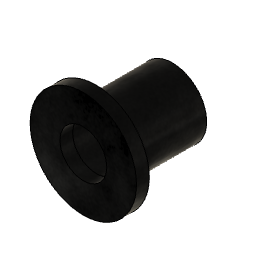
aa FINAL MODEL (Autodesk Fusion 360 archive; units mm, degrees)
design "Black bolt filler for flange"
Autodesk Fusion 360 part; units mm, degrees
note: some values were not read from the file. Chosen so that the rebuilt part matches the saved one: which bodies a step acts on; which face or edge a step refers to; how an offset face is resized.
sketch "Sketch1" plane through (0, 0, 0) normal (0, 1, 0) x (1, 0, 0)
  circle A0 centre (0, 0) radius 12.5
  dimension "d1" = 25
  constraint coincident A0.centre origin
  measures "d1" diameter of A0
extrude "Extrude1" add sketch "Sketch1" along normal blind 3 makes body 1
cylinder "CylinderPrimitive1" add diameter 16 height 18 placed x (1, 0, 0) y (0, 0, -1) z (0, 1, 0) at (0, 3, 0) separate body makes body 2
cylinder "CylinderPrimitive2" cut diameter 11 height -30 placed x (1, 0, 0) y (0, 0, -1) z (0, 1, 0) at (0, 21, 0) bodies 1 2

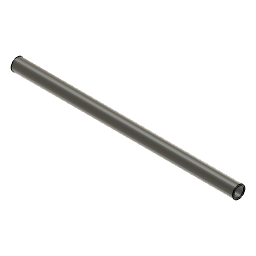
design "Pipe F"
Autodesk Fusion 360 part; units mm, degrees
sketch "Sketch1" plane through (0, 0, 0) normal (0, 1, 0) x (1, 0, 0)
  line L0 (-120, 0) -> (743.6, 0)
  dimension "d1" = 863.6
  constraint horizontal L0
  measures "d1" distance of L0.start L0.end
pipe "Pipe1" add diameter 48 wall 5 path "Sketch1" along L0

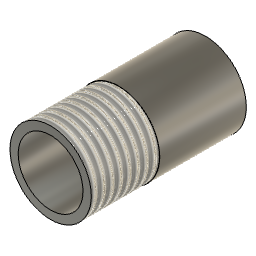
design "Short Piece for Tube"
Autodesk Fusion 360 part; units mm, degrees
sketch "Sketch1" plane through (0, 0, 0) normal (0, 1, 0) x (1, 0, 0)
  circle A0 centre (0, 0) radius 24
  circle A1 centre (0, 0) radius 19
  dimension "d1" = 48
  dimension "d2" = 38
  constraint coincident A0.centre A1.centre
  measures "d1" diameter of A0
  measures "d2" diameter of A1
extrude "Extrude1" add sketch "Sketch1" along normal blind 50.8 makes body 1
sketch "Sketch2" plane through (0, 0, 0) normal (0, -1, 0) x (1, 0, 0)
  circle A0 centre (0, 0) radius 19
  circle A1 centre (0, 0) radius 24
  circle A2 centre (0, 0) radius 24
  circle A3 centre (0, 0) radius 19
  dimension "d5" = 48
  dimension "d6" = 38
  constraint coincident A0.centre A1.centre
  measures "d5" diameter of A2
  measures "d6" diameter of A3
extrude "Extrude2" add sketch "Sketch2" along normal blind 40 bodies 1
sketch "Sketch4" plane through (0, 0, 0) normal (1, 0, 0) x (0, 1, 0)
  line L0 (0, 27) -> (0, -28)
  line L1 (-40, 24) -> (-40, -24)
  dimension "d10" = 40
  constraint vertical L0
  measures "d10" distance of L0 L1
split "Split2" by curves path "Sketch4" along L0 bodies 1 makes body 2 at (23.8807, -13.3333, -2.3896)
thread "Thread1" "ISO Metric profile 48.0 M48x5 M48x5 6g" major diameter 47.664 minor diameter 41.9335 pitch 5 angle 60 resizes the face on face at (23.8807, -13.3333, -2.3896) on bodies 2

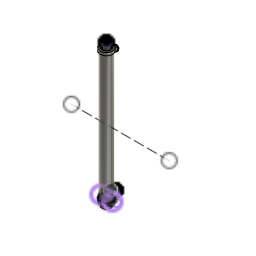
design "Heat Exchange"
Autodesk Fusion 360 part; units mm, degrees
sketch "Sketch1" plane through (0, 0, 0) normal (0, 0, 1) x (1, 0, 0)
  circle A0 centre (0, 0) radius 40
  dimension "d1" = 80
  constraint coincident A0.centre origin
  measures "d1" diameter of A0
extrude "Extrude1" add sketch "Sketch1" along normal blind 914.4 makes body 1
sketch "Sketch2" plane through (0, 0, 914.4) normal (0, 0, 1) x (-1, 0, 0)
  circle A0 centre (0, 0) radius 40
  circle A1 centre (0, 0) radius 44.45
  dimension "d4" = 88.9
  constraint concentric A0 A1
  measures "d4" diameter of A1
extrude "Extrude2" add sketch "Sketch2" along normal blind 20 contours A0 | A1 bodies 1
sketch "Sketch3" plane through (0, 0, 934.4) normal (0, 0, 1) x (-1, 0, 0)
  circle A0 centre (0, 0) radius 44.45
  circle A1 centre (0, 0) radius 29.5
  dimension "d7" = 59
  constraint coincident A0.centre A1.centre
  measures "d7" diameter of A1
extrude "Extrude3" add sketch "Sketch3" along normal blind 31 contours A1 bodies 1
sketch "Sketch4" plane through (0, 0, 965.4) normal (0, 0, 1) x (-1, 0, 0)
  circle A0 centre (0, 0) radius 29.5
  circle A1 centre (0, 0) radius 24
  dimension "d10" = 48
  constraint coincident A0.centre A1.centre
  measures "d10" diameter of A1
extrude "Extrude4" cut sketch "Sketch4" against normal blind 30 contours A1 bodies 1
sketch "Sketch6" plane through (0, 0, 0) normal (0, 0, -1) x (1, 0, 0)
  circle A0 centre (0, 0) radius 40
  circle A1 centre (0, 0) radius 44.45
  dimension "d15" = 88.9
  constraint coincident A0.centre A1.centre
  measures "d15" diameter of A1
extrude "Extrude5" add sketch "Sketch6" along normal blind 20 contours A0 | A1 bodies 1
sketch "Sketch7" plane through (0, 0, -20) normal (0, 0, -1) x (1, 0, 0)
  circle A0 centre (0, 0) radius 44.45
  circle A1 centre (0, 0) radius 22.55
  dimension "d18" = 45.1
  constraint concentric A0 A1
  measures "d18" diameter of A1
ref_plane "WorkPlane2" through (0, 29, 0) normal (0, 1, 0) x (0, 0, 1)
sketch "Sketch10" plane through (0, 29, 0) normal (0, 1, 0) x (1, 0, 0)
  line L0 (22.25, -14.95) -> (22.25, 7.3)
  line L1 (22.25, 7.3) -> (-22.25, 7.3)
  line L2 (-22.25, 7.3) -> (-22.25, -14.95)
  arc A0 (-22.25, -14.95) -> (22.25, -14.95) centre (0, -14.95) ccw
  line L3 (44.45, 20) -> (-44.45, 20)
  point P0 (0, -37.2)
  dimension "d27" = 44.5
  dimension "d28" = 44.5
  dimension "d30" = 12.7
  constraint vertical L0
  constraint perpendicular L0 L1
  constraint perpendicular L1 L2
  constraint tangent L2 A0
  constraint tangent L0 A0
  constraint midpoint A0 P0
  constraint vertical origin A0.centre
  measures "d27" distance of L0.end L1.end
  measures "d28" distance of L1 P0
  measures "d30" distance of L1 L3
extrude "Extrude8" add sketch "Sketch10" along normal blind 28.575 bodies 1
sketch "Sketch11" plane through (0, 57.575, 0) normal (0, 1, 0) x (-1, 0, 0)
  arc A0 (22.25, 14.95) -> (-22.25, 14.95) centre (0, 14.95) ccw
  line L0 (-22.25, 14.95) -> (-22.25, -7.3)
  line L1 (-22.25, -7.3) -> (22.25, -7.3)
  line L2 (22.25, -7.3) -> (22.25, 14.95)
  circle A1 centre (0, 14.95) radius 16
  dimension "d33" = 32
  constraint coincident A0.centre A1.centre
  measures "d33" diameter of A1
extrude "Extrude9" add sketch "Sketch11" along normal blind 5 contours A1 bodies 1
sketch "Sketch12" plane through (0, 0, 0) normal (0, 1, 0) x (1, 0, 0)
  line L0 (450, -457.2) -> (-250, -457.2) construction
  line L1 (44.45, 0) -> (-44.45, 0) construction
  dimension "d36" = 457.2
  constraint horizontal L0
  measures "d36" distance of L0 L1
ref_plane "WorkPlane3" through (0, 0, 458) normal (0, 0, 1) x (1, 0, 0)
mirror "Mirror1" about plane through (0, 0, 458) normal (0, 0, 1) of "Extrude8"
sketch "Sketch13" plane through (0, 62.575, 0) normal (0, 1, 0) x (-1, 0, 0)
  circle A0 centre (0, 14.95) radius 16
  line L0 (0.261, 38.0425) -> (-19.8682, 26.7223)
  line L1 (-19.8682, 26.7223) -> (-20.1292, 3.6298)
  line L2 (-20.1292, 3.6298) -> (-0.261, -8.1425)
  line L3 (-0.261, -8.1425) -> (19.8682, 3.1777)
  line L4 (19.8682, 3.1777) -> (20.1292, 26.2702)
  line L5 (20.1292, 26.2702) -> (0.261, 38.0425)
  point P0 (0, 14.95)
  dimension "d42" = 20
  constraint coincident P0 A0.centre
  measures "d42" distance of P0 L5
extrude "Extrude10" add sketch "Sketch13" along normal blind 4 separate body makes body 2
extrude "Extrude11" add 1 faces at (3.6165, 62.575, 23.0058) along direction (0, 1, 0) blind 7 on bodies 1 bodies 1 2
sketch "Sketch15" plane through (0, 69.575, 0) normal (0, 1, 0) x (-1, 0, 0)
  circle A0 centre (0, 14.95) radius 16
  line L0 (9.7732, 30.6286) -> (-8.6914, 31.2532)
  line L1 (-8.6914, 31.2532) -> (-18.4646, 15.5746)
  line L2 (-18.4646, 15.5746) -> (-9.7732, -0.7286)
  line L3 (-9.7732, -0.7286) -> (8.6914, -1.3532)
  line L4 (8.6914, -1.3532) -> (18.4646, 14.3254)
  line L5 (18.4646, 14.3254) -> (9.7732, 30.6286)
  point P0 (0, 14.95)
  constraint coincident P0 A0.centre
extrude "Extrude13" add sketch "Sketch15" along normal blind 3 bodies 1
mirror "Mirror3" about plane through (0, 0, 458) normal (0, 0, 1) of "Extrude9", "Extrude10", "Extrude11", "Extrude13"
mirror "Mirror4" about plane through (0, 0, 458) normal (0, 0, 1) of "Extrude3"
mirror "Mirror5" about plane through (0, 0, 458) normal (0, 0, 1) of "Extrude4"
thread "Thread1" "ISO Metric profile 48.0 M48x5 M48x5 6H" major diameter 48.5285 minor diameter 42.942 pitch 5 angle 60 resizes the face on face at (-23.9702, 1.1963, 955.4) on bodies 1
thread "Thread2" "ISO Metric profile 48.0 M48x5 M48x5 6H" major diameter 48.5285 minor diameter 42.942 pitch 5 angle 60 resizes the face on face at (-23.9702, 1.1963, -39.4) on bodies 1

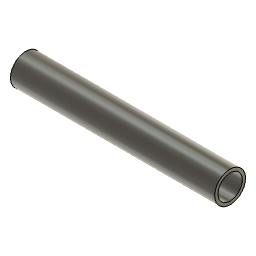
design "Pipe H"
Autodesk Fusion 360 part; units mm, degrees
sketch "Sketch1" plane through (0, 0, 0) normal (0, 1, 0) x (1, 0, 0)
  line L0 (-100, 0) -> (239.7, 0)
  dimension "d1" = 339.7
  constraint horizontal L0
  measures "d1" distance of L0.start L0.end
pipe "Pipe1" add diameter 48 wall 5 path "Sketch1" along L0
extrude "Extrude1" cut 1 faces at (239.7, 2.1363, 22.1732) along direction (-1, 0, 0) blind 21.976

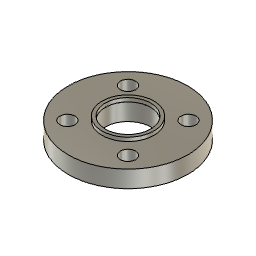
design "1 1/2 Silver Flange"
Autodesk Fusion 360 part; units mm, degrees
sketch "Sketch1" plane through (0, 0, 0) normal (0, 0, 1) x (1, 0, 0)
  circle A0 centre (0, 0) radius 63.5
  dimension "d1" = 127
  constraint coincident A0.centre origin
  measures "d1" diameter of A0
sketch "Sketch2" plane through (0, 0, 18) normal (0, 0, 1) x (-1, 0, 0)
  circle A0 centre (0, 0) radius 63.5
  circle A1 centre (31.1195, -33.1938) radius 8
  circle A2 centre (33.1938, 31.1195) radius 8
  circle A3 centre (-31.1195, 33.1938) radius 8
  circle A4 centre (-33.1938, -31.1195) radius 8
  line L0 (63.467, -2.047) -> (0, 0)
  line L1 (0, 0) -> (-2.047, -63.467)
  line L2 (0, 0) -> (43.4305, -46.3254) construction
  dimension "d4" = 16
  dimension "d8" = 360
  dimension "d9" = 45
  dimension "d10" = 18
  constraint coincident A0 L0.start
  constraint coincident A0.centre L0.end
  constraint coincident A0 L1.end
  constraint perpendicular L0 L1
  constraint coincident A0 L2.end
  constraint coincident A1.centre L2
  measures "d4" diameter of A1
  measures "d9" angle of L0 L2
  measures "d10" distance of A1.centre L2.end
pattern_circular "C-Pattern1" [no effect]
sketch "Sketch3" plane through (0, 0, 18) normal (0, 0, 1) x (-1, 0, 0)
  circle A0 centre (31.1195, -33.1938) radius 8
  circle A1 centre (33.1938, 31.1195) radius 8
  circle A2 centre (-33.1938, -31.1195) radius 8
  circle A3 centre (-31.1195, 33.1938) radius 8
  circle A4 centre (0, 0) radius 63.5
  circle A5 centre (0, 0) radius 24
  dimension "d13" = 48
  constraint coincident A4.centre A5.centre
  measures "d13" diameter of A5
sketch "Sketch4" plane through (0, 0, 18) normal (0, 0, 1) x (-1, 0, 0)
  circle A0 centre (0, 0) radius 24
  circle A1 centre (31.1195, -33.1938) radius 8
  circle A2 centre (33.1938, 31.1195) radius 8
  circle A3 centre (-33.1938, -31.1195) radius 8
  circle A4 centre (-31.1195, 33.1938) radius 8
  circle A5 centre (0, 0) radius 63.5
  circle A6 centre (0, 0) radius 27.5
  dimension "d16" = 55
  constraint coincident A0.centre A5.centre
  measures "d16" diameter of A6
extrude "Extrude4" add sketch "Sketch4" along normal blind 4 contours A6 makes body 1
sketch "Sketch5" plane through (0, 0, 0) normal (0, 0, -1) x (1, 0, 0)
  circle A0 centre (0, 0) radius 24
  circle A1 centre (-31.1195, -33.1938) radius 8
  circle A2 centre (-33.1938, 31.1195) radius 8
  circle A3 centre (33.1938, -31.1195) radius 8
  circle A4 centre (31.1195, 33.1938) radius 8
  arc A5 (0, 63.5) -> (-63.5, 0) centre (0, 0) ccw
  arc A6 (-63.5, 0) -> (0, -63.5) centre (0, 0) ccw
  arc A7 (0, -63.5) -> (63.5, 0) centre (0, 0) ccw
  arc A8 (63.5, 0) -> (0, 63.5) centre (0, 0) ccw
  circle A9 centre (0, 0) radius 35
  dimension "d21" = 70
  constraint coincident A0.centre A5.centre
  measures "d21" diameter of A9
sketch "Sketch6" plane through (0, 0, -5) normal (0, 0, -1) x (1, 0, 0)
  circle A0 centre (0, 0) radius 24
  circle A1 centre (0, 0) radius 35
  circle A2 centre (0, 0) radius 36
  dimension "d24" = 72
  constraint coincident A0.centre A1.centre
  measures "d24" diameter of A2
sketch "Sketch7" plane through (0, 0, 0) normal (0, 0, 1) x (1, 0, 0)
  circle A0 centre (0, 0) radius 63.2942
  constraint coincident A0.centre origin
extrude "Extrude7" cut sketch "Sketch7" along normal blind 18 bodies 1
sketch "Sketch8" plane through (0, 0, 0) normal (0, 0, 1) x (1, 0, 0)
  circle A0 centre (0, 0) radius 63.4217
  constraint coincident A0.centre origin
extrude "Extrude8" add sketch "Sketch8" along normal blind 18 separate body makes body 2
sketch "Sketch9" plane through (0, 0, 18) normal (0, 0, 1) x (-1, 0, 0)
  circle A0 centre (0, 0) radius 63.4217
  circle A1 centre (0, 0) radius 24
  constraint coincident A0.centre A1.centre
extrude "Extrude9" cut sketch "Sketch9" against normal blind 18 contours A1 bodies 2
sketch "Sketch10" plane through (0, 0, 18) normal (0, 0, 1) x (-1, 0, 0)
  circle A0 centre (0, 0) radius 24
  circle A1 centre (0, 0) radius 63.4217
  circle A2 centre (32.1557, -32.1557) radius 8
  circle A3 centre (32.1557, 32.1557) radius 8
  circle A4 centre (-32.1557, 32.1557) radius 8
  circle A5 centre (-32.1557, -32.1557) radius 8
  dimension "d33" = 16
  dimension "d35" = 360
  measures "d33" diameter of A2
extrude "Extrude10" cut sketch "Sketch10" against normal blind 18 contours A2 | A3 | A4 | A5 bodies 2

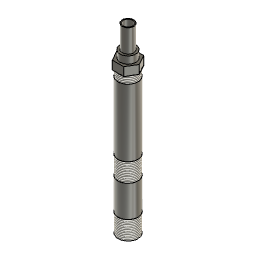
design "valve pipe"
Autodesk Fusion 360 part; units mm, degrees
sketch "Sketch1" plane through (0, 0, 0) normal (0, 0, 1) x (1, 0, 0)
  circle A0 centre (0, 0) radius 7
  dimension "d1" = 14
  constraint coincident A0.centre origin
  measures "d1" diameter of A0
extrude "Extrude1" add sketch "Sketch1" along normal blind 92.1 makes body 1
sketch "Sketch2" plane through (0, 0, 92.1) normal (0, 0, 1) x (-1, 0, 0)
  circle A0 centre (0, 0) radius 7
  line L0 (-7.9997, 0.0678) -> (-4.0586, -6.8941)
  line L1 (-4.0586, -6.8941) -> (3.9411, -6.9619)
  line L2 (3.9411, -6.9619) -> (7.9997, -0.0678)
  line L3 (7.9997, -0.0678) -> (4.0586, 6.8941)
  line L4 (4.0586, 6.8941) -> (-3.9411, 6.9619)
  line L5 (-3.9411, 6.9619) -> (-7.9997, 0.0678)
  dimension "d4" = 8
  constraint coincident A0.centre origin
  measures "d4" distance of L0.start A0.centre
extrude "Extrude2" add sketch "Sketch2" along normal blind 6 separate body contours A0 L0 L1 L2 L3 L4 L5 | A0 L2 L3 | A0 L3 L4 | A0 L1 L2 | A0 L4 L5 | A0 L0 L1 | A0 L0 L5 makes body 2
sketch "Sketch3" plane through (0, 0, 98.1) normal (0, 0, 1) x (-1, 0, 0)
  line L0 (-3.9411, 6.9619) -> (-7.9997, 0.0678)
  line L1 (-7.9997, 0.0678) -> (-4.0586, -6.8941)
  line L2 (-4.0586, -6.8941) -> (3.9411, -6.9619)
  line L3 (3.9411, -6.9619) -> (7.9997, -0.0678)
  line L4 (7.9997, -0.0678) -> (4.0586, 6.8941)
  line L5 (4.0586, 6.8941) -> (-3.9411, 6.9619)
  circle A0 centre (0, 0) radius 5.5
  dimension "d7" = 11
  constraint coincident A0.centre origin
  measures "d7" diameter of A0
extrude "Extrude3" add sketch "Sketch3" along normal blind 5 separate body contours A0 makes body 3
sketch "Sketch4" plane through (0, 0, 103.1) normal (0, 0, 1) x (-1, 0, 0)
  circle A0 centre (0, 0) radius 5.5
  circle A1 centre (0, 0) radius 4
  dimension "d10" = 8
  constraint coincident A0.centre A1.centre
  measures "d10" diameter of A1
extrude "Extrude4" add sketch "Sketch4" along normal blind 16 separate body contours A1 makes body 4
move_body "Move1" bodies 1 4 3 2 to x (1, 0, 0) y (0, 1, 0) z (0, 0, 1) at (0, 0, 4)
extrude "Extrude5" add 1 faces at (1.3617, 1.5871, 4) along direction (0, 0, -1) blind 4 separate body on bodies 1 makes body 5
combine "Combine1" operation add target body 5 tool bodies 1
sketch "Sketch5" plane through (0, 0, 0) normal (0, 1, 0) x (1, 0, 0)
move_body "Move2" bodies 4 5 2 3 to x (1, 0, 0) y (0, 1, 0) z (0, 0, 1) at (0, 0, 4)
extrude "Extrude6" add 1 faces at (2.0592, 1.5871, 4) along direction (0, 0, -1) blind 4 separate body on bodies 5 makes body 6
combine "Combine2" operation add target body 5 tool bodies 6
sketch "Sketch6" plane through (0, 0, 0) normal (0, 1, 0) x (1, 0, 0)
  line L0 (-7, 0) -> (-7, -13)
  line L1 (-7, -13) -> (7, -13)
  dimension "d17" = 13
  constraint vertical L0
  constraint perpendicular L0 L1
  measures "d17" distance of L0.start L0.end
split "Split1" by curves path "Sketch6" along L0 L1 bodies 5 makes body 7 at (-6.9913, 0.3489, 42.0333)
sketch "Sketch7" plane through (0, 0, 0) normal (0, 1, 0) x (1, 0, 0)
  line L0 (-7, -13) -> (-7, -35)
  line L1 (-7, -35) -> (7, -35)
  line L2 (7, -35) -> (7, -40)
  line L3 (7, -40) -> (-7, -40)
  dimension "d18" = 22
  dimension "d19" = 5
  constraint vertical L0
  constraint perpendicular L0 L1
  constraint perpendicular L1 L2
  constraint perpendicular L2 L3
  measures "d18" distance of L0.start L0.end
  measures "d19" distance of L1.end L2.end
split "Split2" by curves path "Sketch7" along L0 L1 L2 L3 bodies 7 makes body 8 at (-6.9913, -0.3489, 27.6667) makes body 9 at (-6.9913, -0.3489, 60.0333)
sketch "Sketch8" plane through (0, 0, 0) normal (0, 1, 0) x (1, 0, 0)
  line L0 (-7, -100) -> (-7, -95)
  line L1 (-7, -95) -> (7, -95)
  dimension "d20" = 5
  constraint vertical L0
  constraint perpendicular L0 L1
  measures "d20" distance of L0.start L0.end
split "Split3" by curves path "Sketch8" along L0 L1 bodies 9 makes body 10 at (-6.9652, -0.697, 58.3333)
thread "Thread1" "ISO Metric profile 14.0 M14x1 M14x1 6g" major diameter 13.884 minor diameter 12.741 pitch 1 angle 60 resizes the face on face at (-6.9652, -0.697, 98.3667) on face at (-6.9913, 0.3489, 8.6667) on face at (-6.9652, -0.697, 36.6667) on bodies 5 7 9
hole "Hole1" at (0, 0, 127.1) direction (0, 0, -1) diameter 6.78 depth 30 tip angle 180 bodies 2 3 4 9
sketch "Sketch9" plane through (0, 0, 0) normal (0, 1, 0) x (1, 0, 0)
  line L0 (-7, -35) -> (-7, -48)
  line L1 (-7, -48) -> (7, -48)
  constraint vertical L0
  constraint perpendicular L0 L1
split "Split4" by curves path "Sketch9" along L0 L1 bodies 10 makes body 11 at (-6.9652, -0.697, 63.6667)
delete_body "RemoveBody1" bodies 10
extrude "Extrude7" add 1 faces at (1.7886, -1.8092, 40) along direction (0, 0, 1) blind 8 on bodies 7 bodies 7 11

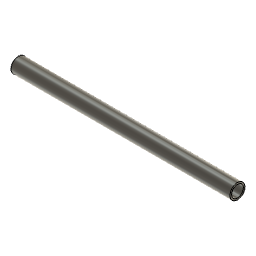
design "Pipe I"
Autodesk Fusion 360 part; units mm, degrees
sketch "Sketch1" plane through (83, 0, 0) normal (1, 0, 0) x (0, 1, 0)
  circle A0 centre (0, 0) radius 19
  circle A1 centre (0, 0) radius 24
  circle A2 centre (0, 0) radius 19
  circle A3 centre (0, 0) radius 24
  circle A4 centre (0, 0) radius 24
  dimension "d1" = 38
  dimension "d2" = 48
  constraint coincident A0.centre A1.centre
  constraint concentric A3 A4
  measures "d1" diameter of A2
  measures "d2" diameter of A4
sketch "Sketch2" plane through (-30, 0, 0) normal (-1, 0, 0) x (0, -1, 0)
  circle A0 centre (0, 0) radius 19
  circle A1 centre (0, 0) radius 24
  circle A2 centre (0, 0) radius 19
  circle A3 centre (0, 0) radius 24
  dimension "d5" = 38
  dimension "d6" = 48
  dimension "d6" = 48
  constraint coincident A0.centre A1.centre
  constraint concentric A0 A3
  measures "d5" diameter of A2
  measures "d6" diameter of A3
extrude "Extrude2" add sketch "Sketch2" along normal blind 698.5

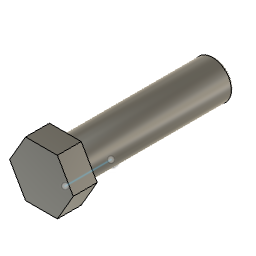
design "pump bolt"
Autodesk Fusion 360 part; units mm, degrees
sketch "Sketch1" plane through (0, 0, 0) normal (0, 1, 0) x (1, 0, 0)
  line L0 (16, 0) -> (8, 13.8564)
  line L1 (8, 13.8564) -> (-8, 13.8564)
  line L2 (-8, 13.8564) -> (-16, 0)
  line L3 (-16, 0) -> (-8, -13.8564)
  line L4 (-8, -13.8564) -> (8, -13.8564)
  line L5 (8, -13.8564) -> (16, 0)
  dimension "d1" = 16
  measures "d1" distance of L0.start origin
extrude "Extrude1" add sketch "Sketch1" against normal blind 12 makes body 1
sketch "Sketch2" plane through (0, 0, 0) normal (0, 1, 0) x (-1, 0, 0)
  line L0 (-8, 13.8564) -> (-16, 0)
  line L1 (-16, 0) -> (-8, -13.8564)
  line L2 (-8, -13.8564) -> (8, -13.8564)
  line L3 (8, -13.8564) -> (16, 0)
  line L4 (16, 0) -> (8, 13.8564)
  line L5 (8, 13.8564) -> (-8, 13.8564)
  circle A0 centre (0, 0) radius 9.5
  dimension "d4" = 19
  constraint coincident A0.centre origin
  measures "d4" diameter of A0
extrude "Extrude2" add sketch "Sketch2" along normal blind 75 separate body contours A0 makes body 2
sketch "Sketch3" plane through (0, 0, 0) normal (1, 0, 0) x (0, 1, 0)
  line L0 (-0.0261, -9.5249) -> (22.9739, -9.5249)
  dimension "d7" = 23
  constraint horizontal L0
  measures "d7" distance of L0.start L0.end
fillet "Fillet1" radius 1 1 edges at (8.8571, 75, -3.4353) on bodies 2

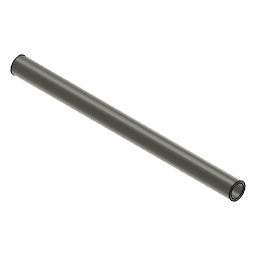
design "Pipe D"
Autodesk Fusion 360 part; units mm, degrees
sketch "Sketch1" plane through (0, 0, 0) normal (0, 1, 0) x (1, 0, 0)
  line L0 (-150, 0) -> (515.16, 0)
  dimension "d1" = 665.16
  constraint horizontal L0
  measures "d1" distance of L0.start L0.end
pipe "Pipe1" add diameter 48 path "Sketch1" along L0
hole "Hole1" at (515.16, 0, 0) direction (-1, 0, 0) diameter 38 depth 700 tip angle 180

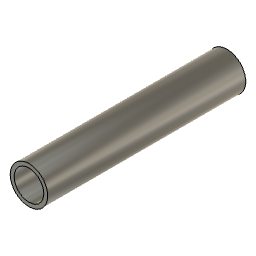
design "Pipe J"
Autodesk Fusion 360 part; units mm, degrees
sketch "Sketch1" plane through (0, 0, 0) normal (0, 1, 0) x (1, 0, 0)
  circle A0 centre (0, 0) radius 24
  circle A1 centre (0, 0) radius 19
  dimension "d1" = 48
  dimension "d2" = 38
  constraint coincident A0.centre A1.centre
  measures "d1" diameter of A0
  measures "d2" diameter of A1
extrude "Extrude1" add sketch "Sketch1" along normal blind 254

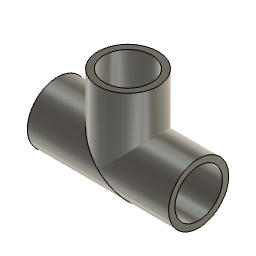
design "T pipe"
Autodesk Fusion 360 part; units mm, degrees
sketch "Sketch1" plane through (0, 0, 0) normal (0, 1, 0) x (1, 0, 0)
  line L0 (-30, 0) -> (83, 0)
  dimension "d1" = 113
  constraint horizontal L0
  measures "d1" distance of L0.start L0.end
pipe "Pipe1" add diameter 48 path "Sketch1" along L0 makes body 1
sketch "Sketch2" plane through (0, 0, 0) normal (0, 1, 0) x (1, 0, 0)
  line L0 (-30, 0) -> (26.5, 0)
  line L1 (26.5, 0) -> (26.5, -58)
  dimension "d6" = 56.5
  dimension "d7" = 58
  constraint horizontal L0
  constraint perpendicular L0 L1
  measures "d6" distance of L0.start L0.end
  measures "d7" distance of L0.end L1.end
pipe "Pipe2" add diameter 48 path "Sketch2" along L1 L0 separate body makes body 2
sketch "Sketch3" plane through (83, 0, 0) normal (1, 0, 0) x (0, 1, 0)
  circle A0 centre (0, 0) radius 24
  circle A1 centre (0, 0) radius 19
  dimension "d12" = 38
  constraint concentric A0 A1
  measures "d12" diameter of A1
extrude "Extrude1" cut sketch "Sketch3" against normal blind 120 contours A1 bodies 1 2
sketch "Sketch4" plane through (0, 0, 58) normal (0, 0, 1) x (-1, 0, 0)
  circle A0 centre (-26.5, 0) radius 24
  circle A1 centre (-26.5, 0) radius 19
  dimension "d15" = 38
  constraint concentric A0 A1
  measures "d15" diameter of A1
extrude "Extrude2" cut sketch "Sketch4" against normal blind 55 contours A1 bodies 1 2

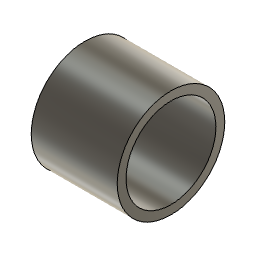
design "pump flange pipe"
Autodesk Fusion 360 part; units mm, degrees
sketch "Sketch1" plane through (0, 0, 0) normal (0, 1, 0) x (1, 0, 0)
  line L0 (0, 0) -> (-48.8, 0)
  dimension "d1" = 48.8
  constraint coincident L0.start origin
  constraint horizontal L0
  measures "d1" distance of L0.start L0.end
pipe "Pipe1" add diameter 61 path "Sketch1" along L0
hole "Hole1" at (0, 0, 0) direction (-1, 0, 0) diameter 51 depth 1000 tip angle 180

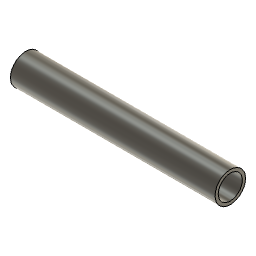
design "Pipe B"
Autodesk Fusion 360 part; units mm, degrees
sketch "Sketch1" plane through (0, 0, 0) normal (0, 1, 0) x (1, 0, 0)
  line L0 (-130, 0) -> (184.3, 0)
  dimension "d1" = 314.3
  constraint horizontal L0
  measures "d1" distance of L0.start L0.end
pipe "Pipe1" add diameter 48 wall 5 path "Sketch1" along L0
extrude "Extrude1" add 1 faces at (-130, 2.1363, 22.1732) along direction (-1, 0, 0) blind 8.356
